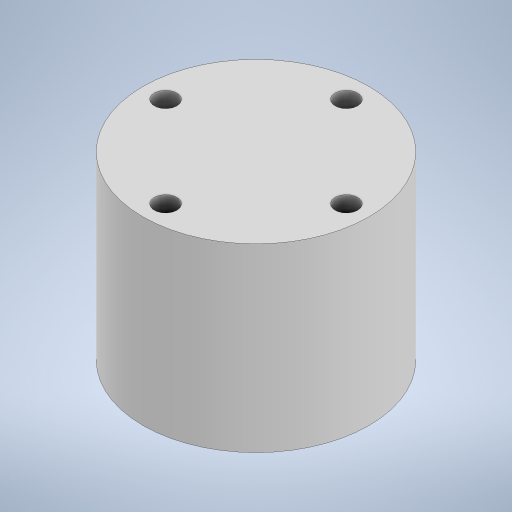
# Autodesk Inventor part: FrontPlatePostNoKey
Saved by Autodesk Inventor 2024 (Build 280153000, 153)
## iProperties
Created: 2024-03-22
Part Number: FrontPlatePostNoKey
Material: Generic
Document SubType Name: Modeling
Designer: yusuf
Density: 1 g/cm^3
Appearance: Default
Author: yusuf
Autodesk Inventor part; units mm, degrees
ref_plane "YZ Plane" through (0, 0, 0) normal (1, 0, 0) x (0, 1, 0)
ref_plane "XZ Plane" through (0, 0, 0) normal (0, 1, 0) x (-1, 0, 0)
ref_plane "XY Plane" through (0, 0, 0) normal (0, 0, 1) x (1, 0, 0)
sketch "Sketch1" plane through (0, 0, 0) normal (0, 1, 0) x (-1, 0, 0)
  circle A0 centre (0, 0) radius 31.75
  dimension "d0" = 63.5
  constraints: 1 centre point, 1 coincident
  measures "d0" diameter of A0
extrude "Extrusion1" add sketch "Sketch1" along normal blind 50.8
sketch "Sketch2" plane through (0, 50.8, 0) normal (0, 1, 0) x (1, 0, 0)
  circle A0 centre (25.4, 0) radius 3.175
  circle A1 centre (0, 25.4) radius 3.175
  circle A2 centre (-25.4, 0) radius 3.175
  circle A3 centre (0, -25.4) radius 3.175
  point P0 (0, 0)
  dimension "d3" = 6.35
  dimension "d6" = 0
  dimension "d7" = 25.4
  dimension "d10" = 360
  constraints: 4 centre point, 9 other
  measures "d3" diameter of A0
  measures "d6" vertical distance of point (0, 0) A0.centre
  measures "d7" distance of point (0, 0) A0.centre
extrude "Extrusion2" cut sketch "Sketch2" against normal blind 50.8
body "Solid1"
